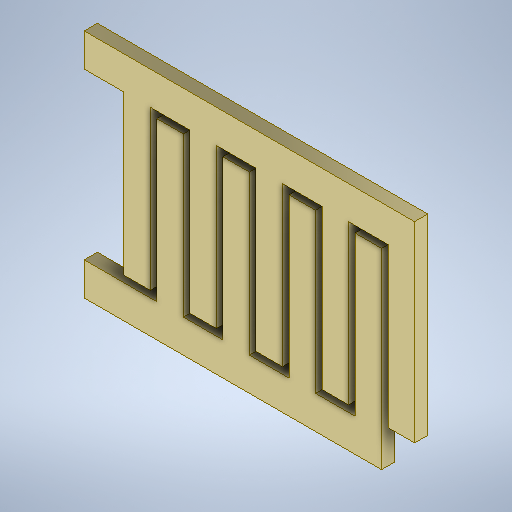
# Autodesk Inventor part: sensor
Saved by Autodesk Inventor 2025.2 (Build 292293000, 293)
## iProperties
Created: 2025-01-21
Part Number: sensor
Material: Generic
Document SubType Name: Modeling
Designer: Tony Dias
Density: 1 g/cm^3
Appearance: Gold - Metal
Author: Tony Dias
Autodesk Inventor part; units mm, degrees
ref_plane "YZ Plane" through (0, 0, 0) normal (1, 0, 0) x (0, 1, 0)
ref_plane "XZ Plane" through (0, 0, 0) normal (0, 1, 0) x (-1, 0, 0)
ref_plane "XY Plane" through (0, 0, 0) normal (0, 0, 1) x (1, 0, 0)
sketch "Sketch1" plane through (0, 0, 0) normal (0, 0, 1) x (1, 0, 0)
  line L0 (-25, 17.5) -> (25, 17.5)
  line L1 (25, -17.5) -> (0, 0) construction
  line L2 (-25, -17.5) -> (25, 17.5) construction
  line L3 (0, 0) -> (-25, 17.5) construction
  line L4 (-25, 17.5) -> (-25, 12.5)
  line L5 (-25, -17.5) -> (-25, -12.5)
  line L6 (25, 17.5) -> (25, -11.5)
  line L7 (25, -11.5) -> (21, -11.5)
  line L8 (21, -11.5) -> (21, 12.5)
  line L9 (21, 12.5) -> (15, 12.5)
  line L10 (15, 12.5) -> (15, -11.5)
  line L11 (15, -11.5) -> (11, -11.5)
  line L12 (11, -11.5) -> (11, 12.5)
  line L13 (11, 12.5) -> (5, 12.5)
  line L14 (5, 12.5) -> (5, -11.5)
  line L15 (5, -11.5) -> (1, -11.5)
  line L16 (1, -11.5) -> (1, 12.5)
  line L17 (1, 12.5) -> (-5, 12.5)
  line L18 (-5, 12.5) -> (-5, -11.5)
  line L19 (-5, -11.5) -> (-9, -11.5)
  line L20 (-9, -11.5) -> (-9, 12.5)
  line L21 (-9, 12.5) -> (-15, 12.5)
  line L22 (-15, 12.5) -> (-15, -11.5)
  line L23 (-15, -11.5) -> (-19, -11.5)
  line L24 (-19, -11.5) -> (-19, 12.5)
  line L25 (-19, 12.5) -> (-25, 12.5)
  line L26 (21, 5.2642) -> (20, 5.2642)
  line L27 (-25, -17.5) -> (20, -17.5)
  line L28 (20, -17.5) -> (20, 11.5)
  line L29 (20, 11.5) -> (16, 11.5)
  line L30 (16, 11.5) -> (16, -12.5)
  line L31 (16, -12.5) -> (10, -12.5)
  line L32 (10, -12.5) -> (10, 11.5)
  line L33 (10, 11.5) -> (6, 11.5)
  line L34 (6, 11.5) -> (6, -12.5)
  line L35 (6, -12.5) -> (0, -12.5)
  line L36 (0, -12.5) -> (0, 11.5)
  line L37 (0, 11.5) -> (-4, 11.5)
  line L38 (-4, 11.5) -> (-4, -12.5)
  line L39 (-4, -12.5) -> (-10, -12.5)
  line L40 (-10, -12.5) -> (-10, 11.5)
  line L41 (-10, 11.5) -> (-14, 11.5)
  line L42 (-14, 11.5) -> (-14, -12.5)
  line L43 (-14, -12.5) -> (-20, -12.5)
  line L44 (-20, -12.5) -> (-25, -12.5)
  dimension "d0" = 35
  dimension "d1" = 50
  dimension "d3" = 5
  dimension "d4" = 5
  dimension "d7" = 29
  dimension "d9" = 4
  dimension "d10" = 24
  dimension "d11" = 6
  dimension "d31" = 1
  dimension "d35" = 4
  dimension "d50" = 24
  constraints: 90 end point, 20 point on line, 7 vertical, 6 horizontal, 6 perpendicular, 2 coincident, 2 midpoint, 1 collinear, 1 parallel
  measures "d0" distance of L2.start L0.start
  measures "d1" distance of L0.start L0.end
  measures "d3" distance of L0.start L4.end
  measures "d4" distance of L5.start L5.end
  measures "d7" distance of L0.end L6.end
  measures "d9" distance of L6.end L7.end
  measures "d10" distance of L7.end L8.end
  measures "d11" distance of L8.end L9.end
  measures "d31" distance of L26.start L26.end
  measures "d35" distance of L28.end L29.end
  measures "d50" distance of L29.end L30.end
extrude "Extrusion1" add sketch "Sketch1" against normal blind 2
body "Solid1"
